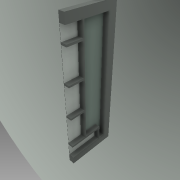
# Autodesk Inventor part: frente salon
Saved by Autodesk Inventor 2015 (Build 190159000, 159)
## iProperties
Created: 2016-01-28
Part Number: frente salon
Material: Generic
Document SubType Name: Modeling
Designer: 172406
Density: 1 g/cm^3
Appearance: Textured - Gray
Author: 172406
Autodesk Inventor part; units mm, degrees
ref_plane "YZ Plane" through (0, 0, 0) normal (1, 0, 0) x (0, 1, 0)
ref_plane "XZ Plane" through (0, 0, 0) normal (0, 1, 0) x (-1, 0, 0)
ref_plane "XY Plane" through (0, 0, 0) normal (0, 0, 1) x (1, 0, 0)
sketch "Sketch1" plane through (0, 0, 0) normal (1, 0, 0) x (0, 1, 0)
  line L0 (0, 0) -> (3600, 0)
  line L1 (3600, 0) -> (3600, -10375)
  line L2 (3600, -10375) -> (0, -10375)
  line L3 (0, -10375) -> (0, 0)
  dimension "d0" = 3600
  dimension "d1" = 10375
  constraints: 8 end point, 2 parallel, 1 horizontal, 1 perpendicular
  measures "d0" distance of L0.start L0.end
  measures "d1" distance of L2.end L0.start
extrude "Extrusion1" add sketch "Sketch1" along normal blind 420
sketch "Sketch2" plane through (420, 0, 0) normal (1, 0, 0) x (0, 0, -1)
  line L0 (597.5, 0) -> (1557.5, 0)
  line L1 (1557.5, 0) -> (1557.5, 1100)
  line L2 (1557.5, 1100) -> (597.5, 1100)
  line L3 (597.5, 1100) -> (597.5, 0)
  line L4 (1697.5, 0) -> (3937.5, 0)
  line L5 (3937.5, 0) -> (3937.5, 1100)
  line L6 (3937.5, 1100) -> (1697.5, 1100)
  line L7 (1697.5, 1100) -> (1697.5, 0)
  line L8 (4077.5, 0) -> (6277.5, 0)
  line L9 (6277.5, 0) -> (6277.5, 1100)
  line L10 (6277.5, 1100) -> (4077.5, 1100)
  line L11 (4077.5, 1100) -> (4077.5, 0)
  line L12 (6417.5, 0) -> (8637.5, 0)
  line L13 (8637.5, 0) -> (8637.5, 1100)
  line L14 (8637.5, 1100) -> (6417.5, 1100)
  line L15 (6417.5, 1100) -> (6417.5, 0)
  line L16 (8777.5, 0) -> (9777.5, 0)
  line L17 (9777.5, 0) -> (9777.5, 2450)
  line L18 (9777.5, 2450) -> (8777.5, 2450)
  line L19 (8777.5, 2450) -> (8777.5, 0)
  line L20 (597.5, 3000) -> (8901.1126, 3000)
  line L21 (8637.5, 2550) -> (8637.5, 1200)
  line L22 (8637.5, 1200) -> (597.5, 1200)
  line L23 (597.5, 1200) -> (597.5, 3000)
  line L24 (8901.1126, 3000) -> (9777.5, 3000)
  line L25 (9777.5, 3000) -> (9777.5, 2550)
  line L26 (9777.5, 2550) -> (8637.5, 2550)
  line L27 (0, 0) -> (10375, 0) projected
  line L28 (0, 0) -> (0, 3600) projected
  line L29 (10375, 0) -> (10375, 3600) projected
  point P0 (1077.5, 0)
  point P1 (2817.5, 0)
  point P2 (5177.5, 0)
  point P3 (7527.5, 0)
  point P4 (9277.5, 0)
  dimension "d4" = 1000
  dimension "d5" = 2450
  dimension "d6" = 140
  dimension "d7" = 140
  dimension "d8" = 140
  dimension "d9" = 140
  dimension "d10" = 960
  dimension "d11" = 2240
  dimension "d12" = 2200
  dimension "d13" = 2220
  dimension "d16" = 100
  dimension "d17" = 3000
  dimension "d18" = 100
  dimension "d19" = 597.5
  dimension "d21" = 1100
  constraints: 54 end point, 13 parallel, 11 point on line, 7 horizontal, 7 perpendicular, 5 midpoint
  measures "d4" distance of L17.end L18.end
  measures "d5" distance of L16.end L17.end
  measures "d6" distance between parallel lines of L13 L19
  measures "d7" distance between parallel lines of L9 L15
  measures "d8" distance between parallel lines of L5 L11
  measures "d9" distance between parallel lines of L1 L7
  measures "d10" distance of L1.end L2.end
  measures "d11" distance of L5.end L6.end
  measures "d12" distance of L9.end L10.end
  measures "d13" distance of L13.end L14.end
  measures "d16" distance between parallel lines of L22 L6
  measures "d17" distance between parallel lines of L20 L27
  measures "d18" distance between parallel lines of L26 L18
  measures "d19" distance between parallel lines of L28 L3
  measures "d21" distance of L2.end L0.start
extrude "Extrusion2" cut sketch "Sketch2" against normal blind 400
body "Solid1"
